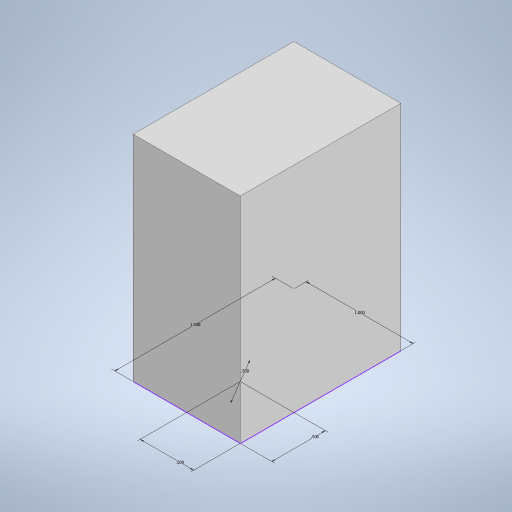
# Autodesk Inventor part: Cylinder
Saved by Autodesk Inventor 2023 (Build 270158000, 158)
## iProperties
Created: 2022-12-28
Part Number: Cylinder
Material: Generic
Document SubType Name: Modeling
Designer: tgr41
Density: 1 g/cm^3
Appearance: Default
Author: tgr41
Autodesk Inventor part; units mm, degrees
ref_plane "YZ Plane" through (0, 0, 0) normal (1, 0, 0) x (0, 1, 0)
ref_plane "XZ Plane" through (0, 0, 0) normal (0, 1, 0) x (-1, 0, 0)
ref_plane "XY Plane" through (0, 0, 0) normal (0, 0, 1) x (1, 0, 0)
sketch "Sketch1" plane through (0, 0, 0) normal (0, 1, 0) x (-1, 0, 0)
  circle A0 centre (3.4811, 6.9947) radius 6.35
  line L0 (-9.2189, 19.6947) -> (16.1811, 19.6947)
  line L1 (16.1811, 19.6947) -> (16.1811, -18.4053)
  line L2 (16.1811, -18.4053) -> (-9.2189, -18.4053)
  line L3 (-9.2189, -18.4053) -> (-9.2189, 19.6947)
  point P0 (0, 0)
  dimension "d0" = 12.7
  dimension "d1" = 25.4
  dimension "d2" = 38.1
  dimension "d3" = 12.7
  dimension "d4" = 12.7
  constraints: 8 end point, 2 parallel, 1 centre point, 1 horizontal, 1 perpendicular
  measures "d0" diameter of A0
  measures "d1" distance of L1.end L2.end
  measures "d2" distance of L0.end L1.end
  measures "d3" distance from line of L3 A0.centre
  measures "d4" distance from line of A0.centre L0
extrude "Extrusion1" add sketch "Sketch1" along normal blind 50.8 contours A0 | L0 L1 L2 L3
extrude "Extrusion4" cut sketch "Sketch1" along normal blind 44.45 contours A0
sketch "Sketch3" plane through (9.2189, 0, -18.4053) normal (0, 0, -1) x (-1, 0, 0)
  line L0 (25.4, 0) -> (0, 0) projected
  line L1 (12.7, 0) -> (12.7, 50.8)
  line L2 (0, 50.8) -> (25.4, 50.8) projected
  circle A0 centre (12.7, 25.4) radius 1.5875
  circle A1 centre (12.7, 38.1) radius 1.5875
  point P0 (9.2189, 0)
  dimension "d23" = 3.175
  dimension "d24" = 3.175
  dimension "d25" = 25.4
  dimension "d26" = 12.7
  constraints: 4 midpoint, 2 centre point, 2 end point, 1 point on line
  measures "d23" diameter of A1
  measures "d24" diameter of A0
  measures "d25" distance from line of L0 A0.centre
  measures "d26" distance of A1.centre point (12.7, 25.4)
extrude "Extrusion5" cut sketch "Sketch3" against normal blind 25.4
body "Solid1"
